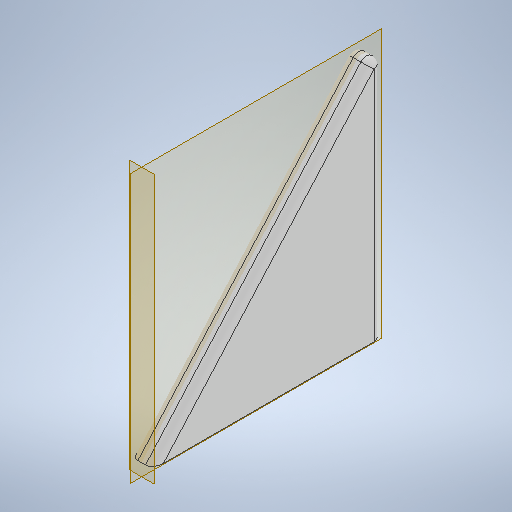
# Autodesk Inventor part: Wing_vertical
Saved by Autodesk Inventor 2027.1 (Build 311270010, 270A)
## iProperties
Created: 2026-09-09
Part Number: Wing_vertical
Material: Generic
Document SubType Name: Modeling
Designer: PWYNNE
Density: 1 g/cm^3
Appearance: Default
Author: PWYNNE
Autodesk Inventor part; units mm, degrees
ref_plane "XZ Plane" through (0, 0, 0) normal (0, 1, 0) x (-1, 0, 0)
sketch "Sketch1" plane through (0, 0, 0) normal (1, 0, 0) x (0, 1, 0)
  line L0 (0, 0) -> (158.3288, -141.2692)
  line L1 (155, -150) -> (0, -150)
  line L2 (0, -150) -> (0, 0)
  arc A0 (155, -150) -> (158.3288, -141.2692) centre (155, -145) ccw
  point P0 (168.114, -150)
  dimension "d1" = 150
  dimension "d2" = 5
  dimension "d3" = 155
  constraints: 6 end point, 2 point on circle, 2 point on line, 2 tangent, 1 centre point, 1 horizontal, 1 perpendicular
  measures "d1" distance of L1.end L0.start
  measures "d2" radius of A0
  measures "d3" distance from line of L2 A0.centre
extrude "Extrusion1" add sketch "Sketch1" along normal mid plane 15
fillet "Fillet1" radius 5 6 edges at (7.5, 159.6719, -146.7813) (7.5, 77.5, -150) (7.5, 79.1644, -70.6346) (-7.5, 159.6719, -146.7813) (-7.5, 77.5, -150) (-7.5, 79.1644, -70.6346)
body "Solid1"
